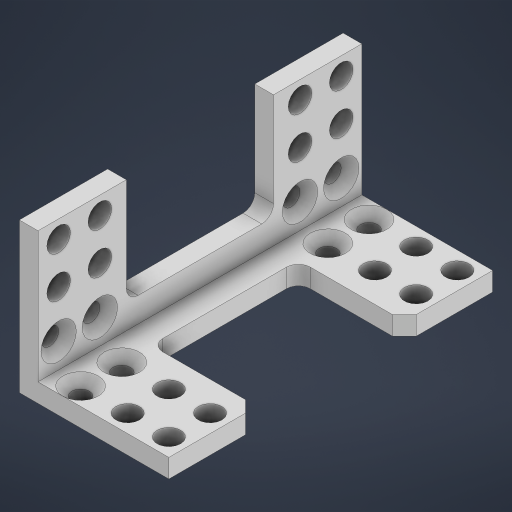
# Autodesk Inventor part: LongL-Bracket
Saved by Autodesk Inventor 2024 (Build 280153000, 153)
## iProperties
Created: 2023-11-23
Part Number: LongL-Bracket
Material: Generic
Document SubType Name: Modeling
Designer: avsar
Density: 1 g/cm^3
Appearance: Default
Author: avsar
Autodesk Inventor part; units mm, degrees
ref_plane "YZ Plane" through (0, 0, 0) normal (1, 0, 0) x (0, 1, 0)
ref_plane "XZ Plane" through (0, 0, 0) normal (0, 1, 0) x (-1, 0, 0)
ref_plane "XY Plane" through (0, 0, 0) normal (0, 0, 1) x (1, 0, 0)
sketch "Sketch1" plane through (0, 0, 0) normal (0, 0, 1) x (1, 0, 0)
  line L0 (0, 0) -> (50.8, 0)
  line L1 (0, 0) -> (0, 50.8)
  line L2 (6.35, 50.8) -> (6.35, 6.35)
  line L3 (6.35, 6.35) -> (50.8, 6.35)
  line L4 (0, 50.8) -> (6.35, 50.8)
  line L5 (50.8, 6.35) -> (50.8, 0)
  dimension "d0" = 50.8
  dimension "d1" = 50.8
  dimension "d2" = 6.35
  constraints: 12 end point, 2 horizontal, 1 perpendicular, 1 vertical, 1 other
  measures "d0" distance of L0.start L0.end
  measures "d1" distance of L0.start L1.end
  measures "d2" distance between parallel lines of L1 L2
extrude "Extrusion1" add sketch "Sketch1" along normal mid plane 110
sketch "Sketch9" plane through (6.35, 6.35, 55) normal (1, 0, 0) x (0, 0, -1)
  line L0 (30, 44.45) -> (80, 44.45)
  line L1 (80, 44.45) -> (80, 8.45)
  line L2 (80, 8.45) -> (30, 8.45)
  line L3 (30, 8.45) -> (30, 44.45)
  line L4 (110, 44.45) -> (0, 44.45) projected
  point P0 (55, -6.35)
  point P1 (55, 44.45)
  dimension "d140" = 50
  dimension "d141" = 36
  constraints: 8 end point, 2 midpoint, 2 parallel, 1 horizontal, 1 perpendicular
  measures "d140" distance of L1.end L2.end
  measures "d141" distance between parallel lines of L0 L2
extrude "Extrusion8" cut sketch "Sketch9" against normal through all
sketch "Sketch8" plane through (6.35, 6.35, 55) normal (1, 0, 0) x (0, 0, -1)
  circle A0 centre (7, 38.45) radius 4
  circle A1 centre (21, 38.45) radius 4
  line L0 (0, 0) -> (0, 44.45) construction
  line L1 (110, 44.45) -> (0, 44.45) construction
  circle A2 centre (7, 24.45) radius 4
  circle A3 centre (21, 24.45) radius 4
  line L2 (55, 44.45) -> (55, 8.45) construction
  line L3 (30, 8.45) -> (80, 8.45) construction
  circle A4 centre (103, 38.45) radius 4
  circle A5 centre (89, 38.45) radius 4
  circle A6 centre (103, 24.45) radius 4
  circle A7 centre (89, 24.45) radius 4
  circle A8 centre (7, 8.45) radius 3
  circle A9 centre (21, 8.45) radius 3
  circle A10 centre (103, 8.45) radius 3
  circle A11 centre (89, 8.45) radius 3
  point P0 (55, -6.35)
  dimension "d135" = 8
  dimension "d136" = 8
  dimension "d137" = 7
  dimension "d138" = 6
  dimension "d139" = 14
  dimension "d146" = 14
  dimension "d160" = 6
  dimension "d161" = 16
  dimension "d162" = 6
  constraints: 12 centre point, 6 symmetric about line, 2 end point, 2 horizontal alignment, 2 midpoint, 2 vertical alignment, 1 vertical, 10 other
  measures "d135" diameter of A0
  measures "d136" diameter of A1
  measures "d137" distance from line of L0 A0.centre
  measures "d138" distance from line of L1 A0.centre
  measures "d139" distance of A1.centre A0.centre
  measures "d146" distance of A0.centre A2.centre
  measures "d160" diameter of A8
  measures "d161" distance of A2.centre A8.centre
  measures "d162" diameter of A9
extrude "Extrusion9" cut sketch "Sketch8" against normal through all
hole "Hole2" at (6.35, 14.8, 48) at (6.35, 14.8, 34) at (6.35, 14.8, -34) at (6.35, 14.8, -48) direction (-1, 0, 0) diameter 6 end through all countersink diameter 12 countersink angle 90
sketch "Sketch10" plane through (6.35, 6.35, 55) normal (0, 1, 0) x (1, 0, 0)
  circle A0 centre (38.45, 6) radius 4
  line L0 (44.45, 0) -> (0, 0) construction
  line L1 (44.45, 110) -> (44.45, 0) construction
  circle A1 centre (38.45, 20) radius 4
  circle A2 centre (24.45, 6) radius 4
  circle A3 centre (24.45, 20) radius 4
  circle A4 centre (8.45, 6) radius 3
  circle A5 centre (8.45, 20) radius 3
  line L2 (0, 110) -> (0, 0) construction
  line L3 (0, 55) -> (44.45, 55) construction
  circle A6 centre (38.45, 104) radius 4
  circle A7 centre (38.45, 90) radius 4
  circle A8 centre (24.45, 104) radius 4
  circle A9 centre (24.45, 90) radius 4
  circle A10 centre (8.45, 104) radius 3
  circle A11 centre (8.45, 90) radius 3
  point P0 (-6.35, 55)
  dimension "d170" = 8
  dimension "d171" = 6
  dimension "d172" = 6
  dimension "d173" = 8
  dimension "d174" = 14
  dimension "d177" = 14
  dimension "d182" = 6
  dimension "d183" = 16
  dimension "d184" = 6
  constraints: 12 centre point, 6 symmetric about line, 2 end point, 2 horizontal alignment, 2 midpoint, 2 vertical alignment, 1 horizontal, 10 other
  measures "d170" diameter of A0
  measures "d171" distance from line of L0 A0.centre
  measures "d172" distance from line of L1 A0.centre
  measures "d173" diameter of A1
  measures "d174" distance of A1.centre A0.centre
  measures "d177" distance of A0.centre A2.centre
  measures "d182" diameter of A4
  measures "d183" distance of A2.centre A4.centre
  measures "d184" diameter of A5
extrude "Extrusion10" cut sketch "Sketch10" against normal through all
hole "Hole3" at (14.8, 6.35, 49) at (14.8, 6.35, 35) at (14.8, 6.35, -35) at (14.8, 6.35, -49) direction (0, -1, 0) diameter 6 end through all countersink diameter 12 countersink angle 90
sketch "Sketch11" plane through (6.35, 6.35, 55) normal (0, 1, 0) x (1, 0, 0)
  line L0 (44.45, 110) -> (44.45, 0) construction
  line L1 (44.45, 80) -> (8.45, 80)
  line L2 (8.45, 80) -> (8.45, 30)
  line L3 (8.45, 30) -> (44.45, 30)
  line L4 (44.45, 30) -> (44.45, 80)
  line L5 (0, 80) -> (0, 30) construction
  point P0 (-6.35, 55)
  dimension "d194" = 36
  constraints: 8 end point, 2 horizontal alignment, 2 parallel, 1 horizontal, 1 perpendicular, 1 point on line
  measures "d194" distance of L2.end L3.end
extrude "Extrusion11" cut sketch "Sketch11" against normal through all
chamfer "Chamfer1" distance 4 angle 45 2 edges at (50.8, 3.175, 25) (50.8, 3.175, -25)
fillet "Fillet1" radius 4 2 edges at (14.8, 3.175, -25) (14.8, 3.175, 25)
fillet "Fillet2" radius 4 2 edges at (3.175, 14.8, 25) (3.175, 14.8, -25)
body "Solid1"
